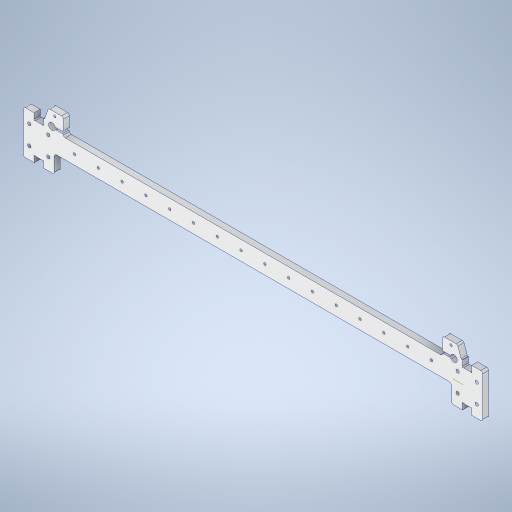
# Autodesk Inventor part: Gantry Bar
Saved by Autodesk Inventor 2024 (Build 280153000, 153)
## iProperties
Created: 2024-08-05
Part Number: Gantry Bar
Material: Aluminum 6061
Document SubType Name: Modeling
Designer: Ishaan
Density: 2.7 g/cm^3
Appearance: Aluminum - Flat
Author: Ishaan
Autodesk Inventor part; units mm, degrees
ref_plane "YZ Plane" through (0, 0, 0) normal (1, 0, 0) x (0, 1, 0)
sketch "Sketch1" plane through (0, 0, 0) normal (0, 0, 1) x (1, 0, 0)
  line L0 (-225, 0) -> (225, 0) construction
  line L1 (-211.5, -16.2) -> (-238.5, -16.2)
  line L2 (-238.5, -16.2) -> (-238.5, 16.2)
  line L3 (-238.5, 16.2) -> (-211.5, 16.2)
  line L4 (-211.5, 16.2) -> (-211.5, -16.2)
  line L5 (-211.5, -16.2) -> (-238.5, 16.2) construction
  line L6 (-238.5, -16.2) -> (-211.5, 16.2) construction
  line L7 (211.5, -16.2) -> (238.5, -16.2)
  line L8 (238.5, -16.2) -> (238.5, 16.2)
  line L9 (238.5, 16.2) -> (211.5, 16.2)
  line L10 (211.5, 16.2) -> (211.5, -16.2)
  line L11 (211.5, -16.2) -> (238.5, 16.2) construction
  line L12 (238.5, -16.2) -> (211.5, 16.2) construction
  line L13 (211.5, -3.8) -> (-211.5, -3.8)
  line L14 (-211.5, -3.8) -> (-211.5, 16.2)
  line L15 (-211.5, 16.2) -> (211.5, 16.2)
  line L16 (211.5, 16.2) -> (211.5, -3.8)
  line L17 (211.5, -3.8) -> (-211.5, 16.2) construction
  line L18 (-211.5, -3.8) -> (211.5, 16.2) construction
  point P0 (0, 0)
  point P1 (0, 0)
  point P2 (0, 6.2)
  point P3 (-211.5, -3.8)
  point P4 (-211.5, 16.2)
  dimension "d0" = 450
  dimension "d1" = 27
  dimension "d2" = 32.4
  dimension "d3" = 20
  constraints: 38 end point, 7 midpoint, 7 parallel, 4 collinear, 4 horizontal, 3 perpendicular, 1 coincident
  measures "d0" distance of L0.start L0.end
  measures "d1" distance of L2.end L3.end
  measures "d2" distance of L1.end L2.end
  measures "d3" distance between parallel lines of L13 L15
extrude "Extrusion1" add sketch "Sketch1" along normal blind 6.35
sketch "Sketch2" plane through (0, 0, 6.35) normal (0, 0, 1) x (1, 0, 0)
  line L0 (-215, -10) -> (-235, -10) construction
  line L1 (-235, -10) -> (-235, 10) construction
  line L2 (-235, 10) -> (-215, 10) construction
  line L3 (-215, 10) -> (-215, -10) construction
  line L4 (-215, -10) -> (-235, 10) construction
  line L5 (-235, -10) -> (-215, 10) construction
  line L6 (235, -10) -> (215, -10) construction
  line L7 (215, -10) -> (215, 10) construction
  line L8 (215, 10) -> (235, 10) construction
  line L9 (235, 10) -> (235, -10) construction
  line L10 (235, -10) -> (215, 10) construction
  line L11 (215, -10) -> (235, 10) construction
  point P0 (0, 0)
  point P1 (-225, 0)
  point P2 (225, 0)
  point P3 (-225, 0)
  point P4 (225, 0)
  dimension "d8" = 20
  dimension "d9" = 20
  dimension "d10" = 20
  dimension "d11" = 20
  constraints: 24 end point, 10 coincident, 4 midpoint, 4 parallel, 2 horizontal, 2 perpendicular
  measures "d8" distance of L1.end L2.end
  measures "d9" distance of L0.end L1.end
  measures "d10" distance of L7.end L8.end
  measures "d11" distance of L6.end L7.end
hole "Hole1" at (-235, 10, 6.35) at (-215, 10, 6.35) at (-215, -10, 6.35) at (-235, -10, 6.35) at (215, 10, 6.35) at (235, 10, 6.35) at (235, -10, 6.35) at (215, -10, 6.35) direction (0, 0, -1) diameter 3.3 end through all
sketch "Sketch3" plane through (0, 0, 6.35) normal (0, 0, 1) x (1, 0, 0)
  circle A0 centre (215, -10) radius 1.65 projected
  circle A1 centre (235, -10) radius 1.65 projected
  circle A2 centre (235, 10) radius 1.65 projected
  circle A3 centre (215, 10) radius 1.65 projected
  circle A4 centre (-235, -10) radius 1.65 projected
  circle A5 centre (-215, -10) radius 1.65 projected
  circle A6 centre (-215, 10) radius 1.65 projected
  circle A7 centre (-235, 10) radius 1.65 projected
  line L0 (-238.5, 16.2) -> (-238.5, -16.2) projected
  line L1 (-238.5, -16.2) -> (-211.5, -16.2) projected
  line L2 (-211.5, -16.2) -> (-211.5, -3.8) projected
  line L3 (-211.5, -3.8) -> (211.5, -3.8) projected
  line L4 (211.5, -3.8) -> (211.5, -16.2) projected
  line L5 (211.5, -16.2) -> (238.5, -16.2) projected
  line L6 (238.5, -16.2) -> (238.5, 16.2) projected
  line L7 (238.5, 16.2) -> (-238.5, 16.2) projected
  line L8 (215, 10) -> (235, -10) construction
  line L9 (-235, -10) -> (-215, 10) construction
  line L10 (-208.8, -16.2) -> (-241.2, -16.2)
  line L11 (-241.2, -16.2) -> (-241.2, 16.2)
  line L12 (-241.2, 16.2) -> (-208.8, 16.2)
  line L13 (-208.8, 16.2) -> (-208.8, -16.2)
  line L14 (-208.8, -16.2) -> (-241.2, 16.2) construction
  line L15 (-241.2, -16.2) -> (-208.8, 16.2) construction
  line L16 (241.2, -16.2) -> (208.8, -16.2)
  line L17 (208.8, -16.2) -> (208.8, 16.2)
  line L18 (208.8, 16.2) -> (241.2, 16.2)
  line L19 (241.2, 16.2) -> (241.2, -16.2)
  line L20 (241.2, -16.2) -> (208.8, 16.2) construction
  line L21 (208.8, -16.2) -> (241.2, 16.2) construction
  point P0 (0, 0)
  point P1 (-225, 0)
  point P2 (225, 0)
  point P3 (238.5, -16.2)
  point P4 (208.8, -3.8)
  point P5 (211.5, -16.2)
  point P6 (-208.8, -3.8)
  point P7 (-211.5, -16.2)
  point P8 (-238.5, -16.2)
  dimension "d19" = 6.2
  dimension "d20" = 6.2
  dimension "d22" = 6.2
  constraints: 28 end point, 6 midpoint, 4 parallel, 2 horizontal, 2 perpendicular, 1 collinear
  measures "d19" distance from line of A7.centre L12
  measures "d20" distance from line of A7.centre L11
  measures "d22" distance from line of L19 A2.centre
extrude "Extrusion2" add sketch "Sketch3" against normal up to surface (6.35 mm away) contours L0 L10 L11 L12 | L2 L3 L13 L10 | L18 L19 L16 L6 | L3 L4 L16 L17
sketch "Sketch4" plane through (0, 0, 6.35) normal (0, 0, 1) x (1, 0, 0)
  line L0 (-241.2, -16.2) -> (-208.8, -16.2) projected
  line L1 (-208.8, -16.2) -> (-208.8, -3.8) projected
  line L2 (-208.8, -3.8) -> (208.8, -3.8) projected
  line L3 (208.8, -3.8) -> (208.8, -16.2) projected
  line L4 (208.8, -16.2) -> (241.2, -16.2) projected
  line L5 (241.2, -16.2) -> (241.2, 16.2) projected
  line L6 (241.2, 16.2) -> (-241.2, 16.2) projected
  line L7 (-241.2, 16.2) -> (-241.2, -16.2) projected
  line L8 (-187.5, 6.2) -> (187.5, 6.2) construction
  line L9 (-208.8, -3.8) -> (208.8, -3.8) construction
  line L10 (0, -3.8) -> (0, 16.2) construction
  point P0 (-162.5, 6.2)
  point P1 (-137.5, 6.2)
  point P2 (-112.5, 6.2)
  point P3 (-87.5, 6.2)
  point P4 (-62.5, 6.2)
  point P5 (-37.5, 6.2)
  point P6 (-12.5, 6.2)
  point P7 (12.5, 6.2)
  point P8 (37.5, 6.2)
  point P9 (62.5, 6.2)
  point P10 (87.5, 6.2)
  point P11 (112.5, 6.2)
  point P12 (137.5, 6.2)
  point P13 (162.5, 6.2)
  point P14 (0, 6.2)
  dimension "d41" = 25
  constraints: 4 end point, 4 midpoint, 2 horizontal, 15 other
  measures "d41" distance of L8.start point (-162.5, 6.2)
hole "Hole2" at (187.5, 6.2, 6.35) at (162.5, 6.2, 6.35) at (137.5, 6.2, 6.35) at (112.5, 6.2, 6.35) at (87.5, 6.2, 6.35) at (62.5, 6.2, 6.35) at (37.5, 6.2, 6.35) at (12.5, 6.2, 6.35) at (-12.5, 6.2, 6.35) at (-37.5, 6.2, 6.35) at (-62.5, 6.2, 6.35) at (-87.5, 6.2, 6.35) at (-112.5, 6.2, 6.35) at (-137.5, 6.2, 6.35) at (-162.5, 6.2, 6.35) at (-187.5, 6.2, 6.35) direction (0, 0, -1) diameter 2.459 end through all thread size "M3x0.5" class "6H" standard "ANSI Metric M Profile"
sketch "Sketch5" plane through (0, 0, 6.35) normal (0, 0, 1) x (1, 0, 0)
  circle A0 centre (-187.5, 6.2) radius 1.2295 projected
  circle A1 centre (-162.5, 6.2) radius 1.2295 projected
  circle A2 centre (-137.5, 6.2) radius 1.2295 projected
  circle A3 centre (-112.5, 6.2) radius 1.2295 projected
  circle A4 centre (-87.5, 6.2) radius 1.2295 projected
  circle A5 centre (-62.5, 6.2) radius 1.2295 projected
  circle A6 centre (-37.5, 6.2) radius 1.2295 projected
  circle A7 centre (-12.5, 6.2) radius 1.2295 projected
  circle A8 centre (12.5, 6.2) radius 1.2295 projected
  circle A9 centre (37.5, 6.2) radius 1.2295 projected
  circle A10 centre (62.5, 6.2) radius 1.2295 projected
  circle A11 centre (87.5, 6.2) radius 1.2295 projected
  circle A12 centre (112.5, 6.2) radius 1.2295 projected
  circle A13 centre (137.5, 6.2) radius 1.2295 projected
  circle A14 centre (162.5, 6.2) radius 1.2295 projected
  circle A15 centre (187.5, 6.2) radius 1.2295 projected
  circle A16 centre (215, -10) radius 1.65 projected
  circle A17 centre (235, -10) radius 1.65 projected
  circle A18 centre (235, 10) radius 1.65 projected
  circle A19 centre (215, 10) radius 1.65 projected
  circle A20 centre (-235, -10) radius 1.65 projected
  circle A21 centre (-215, -10) radius 1.65 projected
  circle A22 centre (-215, 10) radius 1.65 projected
  circle A23 centre (-235, 10) radius 1.65 projected
  line L0 (-241.2, -16.2) -> (-208.8, -16.2) projected
  line L1 (-208.8, -16.2) -> (-208.8, -3.8) projected
  line L2 (-208.8, -3.8) -> (208.8, -3.8) projected
  line L3 (208.8, -3.8) -> (208.8, -16.2) projected
  line L4 (208.8, -16.2) -> (241.2, -16.2) projected
  line L5 (241.2, -16.2) -> (241.2, 16.2) projected
  line L6 (241.2, 16.2) -> (-241.2, 16.2) projected
  line L7 (-241.2, 16.2) -> (-241.2, -16.2) projected
  line L8 (241.2, 16.2) -> (199.2, 16.2)
  line L9 (199.2, 16.2) -> (199.2, 34.2)
  line L10 (199.2, 34.2) -> (241.2, 34.2)
  line L11 (241.2, 34.2) -> (241.2, 16.2)
  line L12 (241.2, -16.2) -> (241.2, 16.2) projected
  line L13 (199.2, 19.7) -> (211.2, 19.7) construction
  line L14 (199.2, 18.7) -> (211.2, 18.7)
  line L15 (211.2, 20.7) -> (199.2, 20.7)
  arc A24 (199.2, 20.7) -> (199.2, 18.7) centre (199.2, 19.7) ccw
  arc A25 (211.2, 18.7) -> (211.2, 20.7) centre (211.2, 19.7) ccw
  circle A26 centre (211.2, 19.7) radius 3.5
  point P0 (0, 0)
  point P1 (205.2, 19.7)
  point P2 (207.8459, 20.7)
  point P3 (216.2, 16.2)
  point P4 (211.2, 16.2)
  point P5 (207.8459, 18.7)
  point P6 (199.2, 16.2)
  point P7 (199.2, 18.7)
  dimension "d46" = 2
  dimension "d47" = 4.5
  dimension "d48" = 7
  dimension "d49" = 12
  dimension "d50" = 18
  dimension "d51" = 42
  constraints: 16 end point, 4 point on circle, 4 tangent, 3 centre point, 3 parallel, 2 perpendicular, 2 point on line, 1 coincident, 1 collinear, 1 horizontal, 1 midpoint
  measures "d46" distance between parallel lines of L14 L15
  measures "d47" distance between parallel lines of L15 L6
  measures "d48" diameter of A26
  measures "d49" distance of L13.start L13.end
  measures "d50" distance between parallel lines of L6 L10
  measures "d51" distance of L9.end L10.end
extrude "Extrusion3" add sketch "Sketch5" against normal up to surface (6.35 mm away) contours L9 L14 A26 L6 | A26 L15 L9 L10 L11 L6 | A26 L14 A25 L15 | L9 L15 A26 L14 | A26 L15 A25 L14
extrude "Extrusion4" cut sketch "Sketch5" against normal through all contours A26 L14 A25 L15 | L9 L15 A26 L14 | A26 L15 A25 L14
fillet "Fillet1" radius 2 2 edges at (207.8459, 20.7, 3.175) (207.8459, 18.7, 3.175)
mirror "Mirror1" about plane through (0, 0, 0) normal (1, 0, 0) of "Extrusion3", "Extrusion4", "Fillet1"
sketch "Sketch7" plane through (0, 0, 6.35) normal (0, 0, 1) x (1, 0, 0)
  line L0 (241.2, -16.2) -> (241.2, 34.2) projected
  line L1 (241.2, 34.2) -> (199.2, 34.2) projected
  arc A0 (-206.5902, 18.7) -> (-208.2665, 17.7909) centre (-206.5902, 16.7) ccw projected
  arc A1 (-208.2665, 21.6091) -> (-208.2665, 17.7909) centre (-211.2, 19.7) ccw projected
  arc A2 (-208.2665, 21.6091) -> (-206.5902, 20.7) centre (-206.5902, 22.7) ccw projected
  line L2 (-206.5902, 20.7) -> (-199.2, 20.7) projected
  line L3 (-199.2, 34.2) -> (-199.2, 20.7) projected
  line L4 (-241.2, 34.2) -> (-199.2, 34.2) projected
  line L5 (-241.2, 34.2) -> (-241.2, -16.2) projected
  line L6 (-241.2, -16.2) -> (-208.8, -16.2) projected
  line L7 (-208.8, -16.2) -> (-208.8, -3.8) projected
  line L8 (-208.8, -3.8) -> (208.8, -3.8) projected
  line L9 (208.8, -3.8) -> (208.8, -16.2) projected
  line L10 (208.8, -16.2) -> (241.2, -16.2) projected
  line L11 (241.2, -16.2) -> (241.2, 34.2) projected
  line L12 (241.2, 34.2) -> (199.2, 34.2) projected
  line L13 (199.2, 34.2) -> (199.2, 20.7) projected
  line L14 (199.2, 20.7) -> (206.5902, 20.7) projected
  arc A3 (206.5902, 20.7) -> (208.2665, 21.6091) centre (206.5902, 22.7) ccw projected
  arc A4 (208.2665, 17.7909) -> (208.2665, 21.6091) centre (211.2, 19.7) ccw projected
  arc A5 (208.2665, 17.7909) -> (206.5902, 18.7) centre (206.5902, 16.7) ccw projected
  line L15 (206.5902, 18.7) -> (199.2, 18.7) projected
  line L16 (199.2, 18.7) -> (199.2, 16.2) projected
  line L17 (199.2, 16.2) -> (-199.2, 16.2) projected
  line L18 (-199.2, 18.7) -> (-199.2, 16.2) projected
  line L19 (-199.2, 18.7) -> (-206.5902, 18.7) projected
  circle A6 centre (-187.5, 6.2) radius 1.2295 projected
  circle A7 centre (-162.5, 6.2) radius 1.2295 projected
  circle A8 centre (-137.5, 6.2) radius 1.2295 projected
  circle A9 centre (-112.5, 6.2) radius 1.2295 projected
  circle A10 centre (-87.5, 6.2) radius 1.2295 projected
  circle A11 centre (-62.5, 6.2) radius 1.2295 projected
  circle A12 centre (-37.5, 6.2) radius 1.2295 projected
  circle A13 centre (-12.5, 6.2) radius 1.2295 projected
  circle A14 centre (12.5, 6.2) radius 1.2295 projected
  circle A15 centre (37.5, 6.2) radius 1.2295 projected
  circle A16 centre (62.5, 6.2) radius 1.2295 projected
  circle A17 centre (87.5, 6.2) radius 1.2295 projected
  circle A18 centre (112.5, 6.2) radius 1.2295 projected
  circle A19 centre (137.5, 6.2) radius 1.2295 projected
  circle A20 centre (162.5, 6.2) radius 1.2295 projected
  circle A21 centre (187.5, 6.2) radius 1.2295 projected
  circle A22 centre (215, -10) radius 1.65 projected
  circle A23 centre (235, -10) radius 1.65 projected
  circle A24 centre (235, 10) radius 1.65 projected
  circle A25 centre (215, 10) radius 1.65 projected
  circle A26 centre (-235, -10) radius 1.65 projected
  circle A27 centre (-215, -10) radius 1.65 projected
  circle A28 centre (-215, 10) radius 1.65 projected
  circle A29 centre (-235, 10) radius 1.65 projected
  circle A30 centre (211.2, 19.7) radius 7.5 construction
  line L20 (199.2, 27.2) -> (204.2, 27.2)
  line L21 (215, -10) -> (235, 10) construction
  line L22 (229.7625, 22.7) -> (220.2375, 22.7) construction
  line L23 (220.2375, 22.7) -> (220.2375, -22.7) construction
  line L24 (220.2375, -22.7) -> (229.7625, -22.7) construction
  line L25 (229.7625, -22.7) -> (229.7625, 22.7) construction
  line L26 (229.7625, 22.7) -> (220.2375, -22.7) construction
  line L27 (220.2375, 22.7) -> (229.7625, -22.7) construction
  line L28 (213.8, -16.2) -> (216.1658, -22.7)
  line L29 (216.1658, -22.7) -> (233.8342, -22.7)
  line L30 (233.8342, -22.7) -> (236.2, -16.2)
  line L31 (241.2, 34.2) -> (241.2, -16.2) projected
  line L32 (241.2, 16.2) -> (236.2, 16.2)
  line L33 (236.2, 16.2) -> (233.8342, 22.7)
  line L34 (233.8342, 22.7) -> (229.7625, 22.7)
  line L35 (220.2375, 22.7) -> (219, 22.7)
  line L36 (219, 22.7) -> (214.8143, 34.2)
  line L37 (236.2, -16.2) -> (236.2, 16.2) construction
  line L38 (220.2375, -22.7) -> (229.7625, -22.7)
  line L39 (229.7625, -22.7) -> (229.7625, -16.2)
  line L40 (229.7625, -16.2) -> (220.2375, -16.2)
  line L41 (220.2375, -16.2) -> (220.2375, -22.7)
  line L42 (220.2375, 22.7) -> (229.7625, 22.7)
  line L43 (229.7625, 22.7) -> (229.7625, 16.2)
  line L44 (229.7625, 16.2) -> (220.2375, 16.2)
  line L45 (220.2375, 16.2) -> (220.2375, 22.7)
  line L46 (204.2, 27.2) -> (204.2, 34.2)
  line L47 (233.8342, 22.7) -> (241.2, 22.7)
  line L48 (208.8, -16.2) -> (241.2, -16.2) projected
  line L49 (241.2, -16.2) -> (208.8, -16.2)
  line L50 (208.8, -16.2) -> (208.8, -22.7)
  line L51 (208.8, -22.7) -> (241.2, -22.7)
  line L52 (241.2, -22.7) -> (241.2, -16.2)
  point P0 (0, 0)
  point P1 (208.2, 30.2)
  point P2 (225, 0)
  point P3 (236.2, 0)
  point P4 (225, -22.7)
  dimension "d59" = 33
  dimension "d60" = 4
  dimension "d61" = 15
  dimension "d62" = 7
  dimension "d63" = 9.525
  dimension "d64" = 45.4
  dimension "d65" = 6
  dimension "d68" = 5
  dimension "d74" = 110
  dimension "d75" = 4
  dimension "d76" = 110
  constraints: 62 end point, 10 parallel, 8 horizontal, 8 point on line, 5 collinear, 5 midpoint, 5 perpendicular, 3 vertical alignment, 1 centre point, 1 coincident, 1 horizontal alignment, 1 vertical
  measures "d59" distance from line of L0 point (208.2, 30.2)
  measures "d60" distance from line of L1 point (208.2, 30.2)
  measures "d61" diameter of A30
  measures "d62" distance between parallel lines of L1 L20
  measures "d63" distance of L24.end L23.end
  measures "d64" distance of L23.end L22.end
  measures "d65" horizontal distance of L35.end point (225, 0)
  measures "d68" distance from line of L28.start L9
  measures "d74" angle of L28 L10
  measures "d75" distance from line of point (208.2, 30.2) L46
  measures "d76" angle of L30 L10
extrude "Extrusion5" add sketch "Sketch7" against normal up to surface (6.35 mm away) contours L52 L51 L30 L10 | L30 L29 L39 L10 | L41 L29 L28 L10 | L28 L51 L50 L10
extrude "Extrusion6" cut sketch "Sketch7" against normal up to surface (6.35 mm away) contours L47 L34 L42 L35 L36 L1 L0 | L43 L44 L45 L42 | A6 | A7 | A8 | A9 | A10 | A11 | A12 | A13 | A14 | A15 | A16 | A17 | A18 | A19 | A20 | A21 | A22 | A23 | A24 | A25 | A26 | A27 | A28 | A29
mirror "Mirror2" about plane through (0, 0, 0) normal (1, 0, 0) of "Extrusion5", "Extrusion6"
sketch "Sketch8" plane through (0, 0, 6.35) normal (0, 0, 1) x (1, 0, 0)
  line L0 (-229.7625, -16.2) -> (-220.2375, -16.2) projected
  line L1 (-229.7625, -16.2) -> (-229.7625, -22.7) projected
  line L2 (-220.2375, -22.7) -> (-220.2375, -16.2) projected
  line L3 (-208.8, -22.7) -> (-208.8, -3.8) projected
  line L4 (-208.8, -3.8) -> (208.8, -3.8) projected
  line L5 (220.2375, -16.2) -> (229.7625, -16.2) projected
  line L6 (220.2375, -22.7) -> (220.2375, -16.2) projected
  line L7 (229.7625, -16.2) -> (229.7625, -22.7) projected
  line L8 (241.2, -22.7) -> (241.2, 22.7) projected
  line L9 (241.2, 22.7) -> (229.7625, 22.7) projected
  line L10 (229.7625, 22.7) -> (229.7625, 16.2) projected
  line L11 (229.7625, 16.2) -> (220.2375, 16.2) projected
  line L12 (220.2375, 16.2) -> (220.2375, 22.7) projected
  line L13 (220.2375, 22.7) -> (219, 22.7) projected
  line L14 (219, 22.7) -> (214.8143, 34.2) projected
  line L15 (214.8143, 34.2) -> (199.2, 34.2) projected
  line L16 (199.2, 34.2) -> (199.2, 20.7) projected
  line L17 (199.2, 20.7) -> (206.5902, 20.7) projected
  arc A0 (206.5902, 20.7) -> (208.2665, 21.6091) centre (206.5902, 22.7) ccw projected
  arc A1 (208.2665, 17.7909) -> (208.2665, 21.6091) centre (211.2, 19.7) ccw projected
  arc A2 (208.2665, 17.7909) -> (206.5902, 18.7) centre (206.5902, 16.7) ccw projected
  line L18 (206.5902, 18.7) -> (199.2, 18.7) projected
  line L19 (199.2, 18.7) -> (199.2, 16.2) projected
  line L20 (199.2, 16.2) -> (-199.2, 16.2) projected
  line L21 (-199.2, 18.7) -> (-199.2, 16.2) projected
  line L22 (-199.2, 18.7) -> (-206.5902, 18.7) projected
  arc A3 (-206.5902, 18.7) -> (-208.2665, 17.7909) centre (-206.5902, 16.7) ccw projected
  arc A4 (-208.2665, 21.6091) -> (-208.2665, 17.7909) centre (-211.2, 19.7) ccw projected
  arc A5 (-208.2665, 21.6091) -> (-206.5902, 20.7) centre (-206.5902, 22.7) ccw projected
  line L23 (-206.5902, 20.7) -> (-199.2, 20.7) projected
  line L24 (-199.2, 34.2) -> (-199.2, 20.7) projected
  line L25 (-214.8143, 34.2) -> (-199.2, 34.2) projected
  line L26 (-214.8143, 34.2) -> (-219, 22.7) projected
  line L27 (-219, 22.7) -> (-220.2375, 22.7) projected
  line L28 (-220.2375, 22.7) -> (-220.2375, 16.2) projected
  line L29 (-220.2375, 16.2) -> (-229.7625, 16.2) projected
  line L30 (-229.7625, 16.2) -> (-229.7625, 22.7) projected
  line L31 (-229.7625, 22.7) -> (-241.2, 22.7) projected
  circle A6 centre (-235, 10) radius 1.65 projected
  circle A7 centre (-215, 10) radius 1.65 projected
  circle A8 centre (-215, -10) radius 1.65 projected
  circle A9 centre (-235, -10) radius 1.65 projected
  circle A10 centre (215, 10) radius 1.65 projected
  circle A11 centre (235, 10) radius 1.65 projected
  circle A12 centre (235, -10) radius 1.65 projected
  circle A13 centre (215, -10) radius 1.65 projected
  circle A14 centre (187.5, 6.2) radius 1.2295 projected
  circle A15 centre (162.5, 6.2) radius 1.2295 projected
  circle A16 centre (137.5, 6.2) radius 1.2295 projected
  circle A17 centre (112.5, 6.2) radius 1.2295 projected
  circle A18 centre (87.5, 6.2) radius 1.2295 projected
  circle A19 centre (62.5, 6.2) radius 1.2295 projected
  circle A20 centre (37.5, 6.2) radius 1.2295 projected
  circle A21 centre (12.5, 6.2) radius 1.2295 projected
  circle A22 centre (-12.5, 6.2) radius 1.2295 projected
  circle A23 centre (-37.5, 6.2) radius 1.2295 projected
  circle A24 centre (-62.5, 6.2) radius 1.2295 projected
  circle A25 centre (-87.5, 6.2) radius 1.2295 projected
  circle A26 centre (-112.5, 6.2) radius 1.2295 projected
  circle A27 centre (-137.5, 6.2) radius 1.2295 projected
  circle A28 centre (-162.5, 6.2) radius 1.2295 projected
  circle A29 centre (-187.5, 6.2) radius 1.2295 projected
  circle A30 centre (229.3625, -16.6) radius 0.75
  line L32 (-241.2, -22.7) -> (-241.2, 22.7) projected
  line L33 (-229.7625, -22.7) -> (-241.2, -22.7) projected
  line L34 (-208.8, -22.7) -> (-220.2375, -22.7) projected
  line L35 (208.8, -3.8) -> (208.8, -22.7) projected
  line L36 (208.8, -22.7) -> (220.2375, -22.7) projected
  line L37 (229.7625, -22.7) -> (241.2, -22.7) projected
  point P0 (0, 0)
  point P1 (229.7625, -17.2344)
  point P2 (228.7281, -16.2)
  dimension "d77" = 1.5
  dimension "d78" = 0.4
  dimension "d82" = 0.4
  constraints: 1 centre point
  measures "d77" diameter of A30
  measures "d78" distance from line of A30.centre L7
  measures "d82" distance from line of L5 A30.centre
extrude "Extrusion7" cut sketch "Sketch8" against normal through all contours A30 L7 L5 | L5 L7 A30 | A6 | A7 | A8 | A9 | A10 | A11 | A12 | A13 | A14 | A15 | A16 | A17 | A18 | A19 | A20 | A21 | A22 | A23 | A24 | A25 | A26 | A27 | A28 | A29
ref_plane "Work Plane1" through (225, -22.7, 0) normal (-1, 0, 0) x (0, 0, 1)
mirror "Mirror3" about plane through (225, -22.7, 0) normal (-1, 0, 0) of "Extrusion7"
ref_plane "Work Plane2" through (228.7281, 0, 0) normal (0, -1, 0) x (1, 0, 0)
mirror "Mirror4" about plane through (228.7281, 0, 0) normal (0, -1, 0) of "Extrusion7", "Mirror3"
mirror "Mirror5" about plane through (0, 0, 0) normal (1, 0, 0) of "Extrusion7", "Mirror3", "Mirror4"
hole "Hole3" at (208.2, 30.2, 6.35) direction (0, 0, -1) diameter 2.459 end through all thread size "M3x0.5" class "6H" standard "ANSI Metric M Profile"
mirror "Mirror6" about plane through (0, 0, 0) normal (1, 0, 0) of "Hole3"
fillet "Fillet3" radius 2 6 edges at (241.2, 22.7, 3.175) (241.2, -22.7, 3.175) (208.8, -22.7, 3.175) (-208.8, -22.7, 3.175) (-241.2, -22.7, 3.175) (-241.2, 22.7, 3.175)
fillet "Fillet4" radius 3 2 edges at (-208.8, -3.8, 3.175) (208.8, -3.8, 3.175)
fillet "Fillet5" radius 2 2 edges at (199.2, 16.2, 3.175) (-199.2, 16.2, 3.175)
fillet "Fillet6" radius 1 2 edges at (-219, 22.7, 3.175) (219, 22.7, 3.175)
fillet "Fillet7" radius 2 4 edges at (214.8143, 34.2, 3.175) (-199.2, 34.2, 3.175) (-214.8143, 34.2, 3.175) (199.2, 34.2, 3.175)
fillet "Fillet8" radius 1 4 edges at (-199.2, 20.7, 3.175) (-199.2, 18.7, 3.175) (199.2, 20.7, 3.175) (199.2, 18.7, 3.175)
ref_plane "Work Plane3" through (220.2375, 0.8, 0) normal (0, -1, 0) x (1, 0, 0)
equation "\"d20\" = d19"
equation "\"d22\" = d21"
equation "\"d75\" = d60"
equation "\"d76\" = d74"
equation "\"d82\" = d78"
equation "\"d21\" = 6.2"
body "Solid1"
